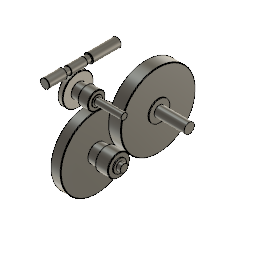
Gearbox Final v12 (Autodesk Fusion 360 design; units mm, degrees)
description: Stage 1
part number: KWG1-R2
description: Layshaft 1
part number: CG1-60R1
description: Stage 2
part number: SSG2-17
description: Layshaft 3
part number: SSG2.5-17
description: Layshaft 2
part number: SSA2-70
description: Stage 3
part number: SS2.5-58
Autodesk Fusion 360 part; units mm, degrees
sketch "Sketch1" plane through (0, 0, 0) normal (0, 1, 0) x (1, 0, 0)
  circle A0 centre (0, 0) radius 9.1
  dimension "d1" = 18.2
  constraint coincident A0.centre origin
  measures "d1" diameter of A0
extrude "Extrude1" add sketch "Sketch1" along normal blind 35 makes body 1
sketch "Sketch2" plane through (0, 35, 0) normal (0, 1, 0) x (-1, 0, 0)
  circle A0 centre (0, 0) radius 9.1
  circle A1 centre (0, 0) radius 6.5
  dimension "d4" = 13
  constraint coincident A0.centre A1.centre
  measures "d4" diameter of A1
extrude "Extrude2" add sketch "Sketch2" along normal blind 10 contours A1 bodies 1
sketch "Sketch3" plane through (0, 45, 0) normal (0, 1, 0) x (-1, 0, 0)
  circle A0 centre (0, 0) radius 6.5
  circle A1 centre (0, 0) radius 8
  dimension "d7" = 16
  constraint coincident A0.centre A1.centre
  measures "d7" diameter of A1
extrude "Extrude3" add sketch "Sketch3" along normal blind 30 contours A0 | A1 bodies 1
sketch "Sketch4" plane through (0, 75, 0) normal (0, 1, 0) x (-1, 0, 0)
  circle A0 centre (0, 0) radius 8
  circle A1 centre (0, 0) radius 6.5
  dimension "d10" = 13
  constraint coincident A0.centre A1.centre
  measures "d10" diameter of A1
extrude "Extrude4" add sketch "Sketch4" along normal blind 10 contours A1 bodies 1
sketch "Sketch5" plane through (0, 85, 0) normal (0, 1, 0) x (-1, 0, 0)
  circle A0 centre (0, 0) radius 6.5
  circle A1 centre (0, 0) radius 9.1
  dimension "d13" = 18.2
  constraint coincident A0.centre A1.centre
  measures "d13" diameter of A1
extrude "Extrude5" add sketch "Sketch5" along normal blind 55 contours A0 | A1 bodies 1
chamfer "Chamfer1" distance 0.5 angle 45 4 edges at (-8.4842, 0, 3.2907) (-8.4842, 35, 3.2907) (8.4842, 85, -3.2907) (8.4842, 140, -3.2907) on bodies 1
sketch "Sketch6" plane through (0, 0, 0) normal (1, 0, 0) x (0, 1, 0)
  circle A0 centre (55, -45) radius 30.06
  circle A1 centre (55, -45) radius 5
  dimension "d17" = 60.12
  dimension "d18" = 10
  constraint concentric A0 A1
  measures "d17" diameter of A0
  measures "d18" diameter of A1
extrude "Extrude6" add sketch "Sketch6" against normal blind 10 separate body makes body 2
sketch "Sketch7" plane through (-10, 0, 0) normal (-1, 0, 0) x (0, -1, 0)
  circle A0 centre (-55, -45) radius 5
  circle A1 centre (-55, -45) radius 30.06
  circle A2 centre (-55, -45) radius 15
  dimension "d21" = 30
  constraint concentric A0 A2
  measures "d21" diameter of A2
extrude "Extrude7" add sketch "Sketch7" along normal blind 10 contours A2 bodies 2
chamfer "Chamfer2" distance 1 angle 45 2 edges at (0, 26.9742, -55.8702) (-10, 26.9742, -34.1298) on bodies 2
chamfer "Chamfer2" distance 0.5 angle 45 3 edges at (0, 50.3384, -43.1919) (-20, 68.9849, -50.4242) (-20, 59.6616, -43.1919) on bodies 2
move_body "Move1" bodies 2 to x (1, 0, 0) y (0, 1, 0) z (0, 0, 1) at (5, 5, 22)
sketch "Sketch8" plane through (5, 0, 0) normal (1, 0, 0) x (0, 1, 0)
  circle A0 centre (60, -23) radius 29.06
  circle A1 centre (60, -23) radius 5.5
  circle A2 centre (60, -23) radius 3
  dimension "d26" = 6
  constraint concentric A0 A2
  measures "d26" diameter of A2
sketch "Sketch11" plane through (0, 0, 0) normal (1, 0, 0) x (0, 1, 0)
  circle A0 centre (0, -50) radius 17
  circle A1 centre (0, -50) radius 6
  dimension "d34" = 34
  dimension "d35" = 12
  constraint concentric A0 A1
  measures "d34" diameter of A0
  measures "d35" diameter of A1
extrude "Extrude10" add sketch "Sketch11" along normal blind 20 separate body makes body 3
sketch "Sketch12" plane through (20, 0, 0) normal (1, 0, 0) x (0, 1, 0)
  circle A0 centre (0, -50) radius 6
  circle A1 centre (0, -50) radius 17
  circle A2 centre (0, -50) radius 14
  dimension "d38" = 28
  constraint concentric A0 A2
  measures "d38" diameter of A2
extrude "Extrude11" add sketch "Sketch12" along normal blind 16 contours A2 bodies 3
chamfer "Chamfer3" distance 0.5 angle 45 3 edges at (36, -13.0526, -55.0626) (36, -5.594, -47.8303) (0, -5.594, -47.8303) on bodies 3
chamfer "Chamfer3" distance 1 angle 45 2 edges at (0, -15.8496, -56.1475) (20, -15.8496, -56.1475) on bodies 3
sketch "Sketch14" plane through (5, 0, 0) normal (1, 0, 0) x (0, 1, 0)
  circle A0 centre (60, -23) radius 29.06
  circle A1 centre (60, -23) radius 5.5
  circle A2 centre (60, -23) radius 5
  dimension "d46" = 10
  constraint concentric A0 A2
  measures "d46" diameter of A2
extrude "Extrude13" add sketch "Sketch14" along normal blind 0 and the other way blind 25 separate body contours A2 makes body 4
sketch "Sketch15" plane through (5, 0, 0) normal (1, 0, 0) x (0, 1, 0)
  circle A0 centre (60, -23) radius 5
  circle A1 centre (60, -23) radius 6
  dimension "d52" = 12
  constraint concentric A0 A1
  measures "d52" diameter of A1
move_body "Move2" bodies 4 to x (1, 0, 0) y (0, 1, 0) z (0, 0, 1) at (43, 0, 0)
sketch "Sketch16" plane through (48, 0, 0) normal (1, 0, 0) x (0, 1, 0)
  circle A0 centre (60, -23) radius 5
  circle A1 centre (60, -23) radius 6
  dimension "d55" = 12
  constraint concentric A0 A1
  measures "d55" diameter of A1
extrude "Extrude15" add sketch "Sketch16" along normal blind 36 contours A0 | A1 bodies 4
move_body "Move3" bodies 4 to x (1, 0, 0) y (0, 1, 0) z (0, 0, 1) at (-43, 0, 0)
move_body "Move4" bodies 3 to x (-1, 0, 0) y (0, 1, 0) z (0, 0, -1) at (41, 60, -73)
sketch "Sketch17" plane through (41, 0, 0) normal (1, 0, 0) x (0, 1, 0)
  circle A0 centre (60, -23) radius 6
  circle A1 centre (60, -23) radius 10
  dimension "d58" = 20
  constraint concentric A0 A1
  measures "d58" diameter of A1
sketch "Sketch18" plane through (0, 0, 0) normal (1, 0, 0) x (0, 1, 0)
  circle A0 centre (0, -150) radius 70
  circle A1 centre (0, -150) radius 9
  dimension "d61" = 140
  dimension "d62" = 18
  constraint concentric A0 A1
  measures "d61" diameter of A0
  measures "d62" diameter of A1
extrude "Extrude17" add sketch "Sketch18" along normal blind 20 separate body makes body 5
move_body "Move5" bodies 5 to x (1, 0, 0) y (0, 1, 0) z (0, 0, 1) at (21, 60, 40)
sketch "Sketch19" plane through (41, 0, 0) normal (1, 0, 0) x (0, 1, 0)
  circle A0 centre (60, -110) radius 9
  circle A1 centre (60, -110) radius 9
  circle A2 centre (60, -110) radius 70
  dimension "d69" = 18
  measures "d69" diameter of A0
extrude "Extrude18" add sketch "Sketch19" along normal blind 0 and the other way blind 30 separate body contours A0 A1 makes body 6
sketch "Sketch20" plane through (0, 0, 0) normal (1, 0, 0) x (0, 1, 0)
  circle A0 centre (0, -300) radius 21.25
  circle A1 centre (0, -300) radius 7.5
  dimension "d74" = 42.5
  dimension "d75" = 15
  constraint concentric A0 A1
  measures "d74" diameter of A0
  measures "d75" diameter of A1
extrude "Extrude19" add sketch "Sketch20" along normal blind 25 separate body makes body 7
sketch "Sketch21" plane through (25, 0, 0) normal (1, 0, 0) x (0, 1, 0)
  circle A0 centre (0, -300) radius 7.5
  circle A1 centre (0, -300) radius 21.25
  circle A2 centre (0, -300) radius 17.5
  dimension "d78" = 35
  constraint concentric A0 A2
  measures "d78" diameter of A2
extrude "Extrude20" add sketch "Sketch21" along normal blind 18 contours A2 bodies 7
chamfer "Chamfer4" distance 0.5 angle 45 3 edges at (0, -6.9925, -297.2879) (43, -16.3157, -306.3283) (43, -6.9925, -297.2879) on bodies 7
chamfer "Chamfer4" distance 1 angle 45 2 edges at (25, -19.812, -307.6843) (0, -19.812, -307.6843) on bodies 7
move_body "Move6" bodies 7 to x (-1, 0, 0) y (0, 1, 0) z (0, 0, -1) at (84, 60, -408.5)
sketch "Sketch22" plane through (0, 0, 0) normal (1, 0, 0) x (0, 1, 0)
  circle A0 centre (0, -325) radius 72.5
  circle A1 centre (0, -325) radius 10
  dimension "d83" = 145
  dimension "d84" = 20
  constraint concentric A0 A1
  measures "d83" diameter of A0
  measures "d84" diameter of A1
extrude "Extrude21" add sketch "Sketch22" along normal blind 25 separate body makes body 8
sketch "Sketch23" plane through (25, 0, 0) normal (1, 0, 0) x (0, 1, 0)
  circle A0 centre (0, -325) radius 10
  circle A1 centre (0, -325) radius 72.5
  circle A2 centre (0, -325) radius 35
  dimension "d87" = 70
  constraint concentric A0 A2
  measures "d87" diameter of A2
extrude "Extrude22" add sketch "Sketch23" along normal blind 12 contours A2 bodies 8
chamfer "Chamfer5" distance 0.5 angle 45 3 edges at (37, -32.6315, -337.6565) (37, -9.3233, -321.3838) (0, -9.3233, -321.3838) on bodies 8
chamfer "Chamfer5" distance 1 angle 45 2 edges at (25, -67.5937, -351.2171) (0, -67.5937, -351.2171) on bodies 8
move_body "Move7" bodies 8 to x (-1, 0, 0) y (0, 1, 0) z (0, 0, -1) at (121, 136.4009, -379.3337)
move_body "Move8" bodies 8 to x (1, 0, 0) y (0, 1, 0) z (0, 0, 1) at (-37, 0, 0)
sketch "Sketch24" plane through (84, 0, 0) normal (1, 0, 0) x (0, 1, 0)
  circle A0 centre (136.4009, -54.3337) radius 10.5
  circle A1 centre (136.4009, -54.3337) radius 71.5
  circle A2 centre (136.4009, -54.3337) radius 10
  dimension "d94" = 20
  constraint concentric A0 A2
  measures "d94" diameter of A2
extrude "Extrude24" add sketch "Sketch24" along normal blind 60 and the other way blind 37 separate body contours A2 makes body 9
move_body "Move9" bodies 6 to x (1, 0, 0) y (0, 1, 0) z (0, 0, 1) at (120, 0, 0)
extrude "Extrude25" cut 1 faces at (131, 62.5872, -107.1538) along direction (1, 0, 0) blind 10 on bodies 6 bodies 6
sketch "Sketch25" plane through (161, 0, 0) normal (1, 0, 0) x (0, 1, 0)
  circle A0 centre (60, -110) radius 9
  circle A1 centre (60, -110) radius 7.5
  dimension "d101" = 15
  constraint concentric A0 A1
  measures "d101" diameter of A1
extrude "Extrude26" add sketch "Sketch25" along normal blind 43 contours A1 bodies 6
sketch "Sketch27" plane through (141, 0, 0) normal (-1, 0, 0) x (0, -1, 0)
  circle A0 centre (-60, -110) radius 9
  circle A1 centre (-60, -110) radius 15
  dimension "d107" = 30
  constraint concentric A0 A1
  measures "d107" diameter of A1
extrude "Extrude28" add sketch "Sketch27" along normal blind 2 contours A0 | A1 bodies 6
move_body "Move10" bodies 7 8 9 to x (1, 0, 0) y (0, 1, 0) z (0, 0, 1) at (0, 0, -1.5)
move_body "Move11" bodies 6 to x (1, 0, 0) y (0, 1, 0) z (0, 0, 1) at (-120, 0, 0)
extrude "Extrude29" add 1 faces at (84, 59.4437, -107.783) along direction (1, 0, 0) blind 10 on bodies 6 bodies 6
sketch "Sketch28" plane through (19, 0, 0) normal (-1, 0, 0) x (0, -1, 0)
  circle A0 centre (-60, -110) radius 15
  circle A1 centre (-60, -110) radius 9
  dimension "d112" = 18
  constraint concentric A0 A1
  measures "d112" diameter of A1
extrude "Extrude30" add sketch "Sketch28" along normal up to surface (39 mm away) contours A1 bodies 6
move_body "Move12" bodies 9 to x (1, 0, 0) y (0, 1, 0) z (0, 0, 1) at (95, 0, 0)
sketch "Sketch29" plane through (142, 0, 0) normal (-1, 0, 0) x (0, -1, 0)
  circle A0 centre (-136.4009, -55.8337) radius 10
  circle A1 centre (-136.4009, -55.8337) radius 15
  dimension "d115" = 30
  constraint concentric A0 A1
  measures "d115" diameter of A1
extrude "Extrude31" add sketch "Sketch29" along normal blind 2 contours A0 | A1 bodies 9
move_body "Move13" bodies 9 to x (1, 0, 0) y (0, 1, 0) z (0, 0, 1) at (-95, 0, 0)
move_body "Move14" bodies 4 to x (1, 0, 0) y (0, 1, 0) z (0, 0, 1) at (130, 0, 0)
sketch "Sketch30" plane through (171, 0, 0) normal (1, 0, 0) x (0, 1, 0)
  circle A0 centre (60, -23) radius 6
  circle A1 centre (60, -23) radius 10
  dimension "d119" = 20
  constraint concentric A0 A1
  measures "d119" diameter of A1
extrude "Extrude32" add sketch "Sketch30" along normal blind 1 contours A0 | A1 bodies 4
move_body "Move15" bodies 4 to x (1, 0, 0) y (0, 1, 0) z (0, 0, 1) at (-130, 0, 0)
sketch "Sketch32" plane through (42, 0, 0) normal (1, 0, 0) x (0, 1, 0)
  circle A0 centre (60, -23) radius 10
  circle A1 centre (60, -23) radius 6
  dimension "d123" = 12
  constraint concentric A0 A1
  measures "d123" diameter of A1
extrude "Extrude33" add sketch "Sketch32" along normal up to surface (52 mm away) contours A1 bodies 4
sketch "Sketch33" plane through (84, 0, 0) normal (1, 0, 0) x (0, 1, 0)
  circle A0 centre (136.4009, -55.8337) radius 10.5
  circle A1 centre (136.4009, -55.8337) radius 71.5
  circle A2 centre (136.4009, -55.8337) radius 20
  circle A3 centre (136.4009, -55.8337) radius 10
  dimension "d126" = 40
  dimension "d127" = 20
  constraint concentric A0 A2
  constraint concentric A2 A3
  measures "d126" diameter of A2
  measures "d127" diameter of A3
extrude "Extrude34" add sketch "Sketch33" along normal blind 2 separate body contours A0 | A2 makes body 10
sketch "Sketch34" plane through (84, 0, 0) normal (1, 0, 0) x (0, 1, 0)
  circle A0 centre (60, -110) radius 8
  circle A1 centre (60, -110) radius 20.25
  circle A2 centre (60, -110) radius 12.5
  circle A3 centre (60, -110) radius 7.5
  dimension "d130" = 25
  dimension "d131" = 15
  constraint concentric A0 A2
  constraint concentric A2 A3
  measures "d130" diameter of A2
  measures "d131" diameter of A3
extrude "Extrude35" add sketch "Sketch34" along normal blind 2 separate body contours A0 | A2 makes body 11
sketch "Sketch35" plane through (-15, 0, 0) normal (-1, 0, 0) x (0, -1, 0)
  circle A0 centre (-60, -23) radius 14.5
  circle A1 centre (-60, -23) radius 5.5
  circle A2 centre (-60, -23) radius 10
  circle A3 centre (-60, -23) radius 5
  dimension "d134" = 20
  dimension "d135" = 10
  constraint concentric A0 A2
  constraint concentric A2 A3
  measures "d134" diameter of A2
  measures "d135" diameter of A3
extrude "Extrude36" add sketch "Sketch35" along normal blind 1 separate body contours A1 | A2 makes body 12
move_body "Move16" bodies 1 to x (1, 0, 0) y (0, 1, 0) z (0, 0, 1) at (0, 0, 15)
copy_body "Body->Comp1" bodies 1 removing the originals makes body 13 in component "Worm "
copy_body "Body->Comp2" bodies 12 removing the originals makes body 14 in component "Fixing "
copy_body "Body->Comp3" bodies 2 removing the originals makes body 15 in component "Wheel"
copy_body "Body->Comp4" bodies 3 removing the originals makes body 16 in component "Spur 17 M2"
copy_body "Body->Comp5" bodies 4 removing the originals makes body 17 in component "Layshaft 1"
copy_body "Body->Comp6" bodies 10 removing the originals makes body 18 in component "Fixing 3"
copy_body "Body->Comp7" bodies 9 removing the originals makes body 19 in component "Layshaft 3"
copy_body "Body->Comp8" bodies 7 removing the originals makes body 20 in component "Spur 17 M2.5"
copy_body "Body->Comp9" bodies 11 removing the originals makes body 21 in component "Fixing 2"
copy_body "Body->Comp10" bodies 5 removing the originals makes body 22 in component "Spur 70 M2"
copy_body "Body->Comp11" bodies 8 removing the originals makes body 23 in component "Spur 58 M2.5"
copy_body "Body->Comp12" bodies 6 removing the originals makes body 24 in component "Layshaft 2"
chamfer "Chamfer1'" distance 1 angle 45 2 edges at (41, -5.2629, -135.3131) (21, -5.2629, -135.3131) on bodies 22 in component "Spur 70 M2"
component "Worm " placed x (1, 0, 0) y (0, 1, 0) z (0, 0, 1) at (0, 0, 0)
component "Fixing " placed x (1, 0, 0) y (0, 1, 0) z (0, 0, 1) at (0, 0, 0)
component "Wheel" placed x (1, 0, 0) y (0, 1, 0) z (0, 0, 1) at (0, 0, 0)
component "Spur 17 M2" placed x (1, 0, 0) y (0, 1, 0) z (0, 0, 1) at (0, 0, 0)
component "Layshaft 1" placed x (1, 0, 0) y (0, 1, 0) z (0, 0, 1) at (0, 0, 0)
component "Fixing 3" placed x (1, 0, 0) y (0, 1, 0) z (0, 0, 1) at (0, 0, 0)
component "Layshaft 3" placed x (1, 0, 0) y (0, 1, 0) z (0, 0, 1) at (0, 0, 0)
component "Spur 17 M2.5" placed x (1, 0, 0) y (0, 1, 0) z (0, 0, 1) at (0, 0, 0)
component "Fixing 2" placed x (1, 0, 0) y (0, 1, 0) z (0, 0, 1) at (0, 0, 0)
component "Spur 70 M2" placed x (1, 0, 0) y (0, 1, 0) z (0, 0, 1) at (0, 0, 0)
component "Spur 58 M2.5" placed x (1, 0, 0) y (0, 1, 0) z (0, 0, 1) at (0, 0, 0)
component "Layshaft 2" placed x (1, 0, 0) y (0, 1, 0) z (0, 0, 1) at (0, 0, 0)
named bodies: "Worm", "Wheel", "Spur 17 M2", "Layshaft 1", "Spur 70 M2", "Layshaft 2", "Spur 17 M2.5", "Spur 58 M2.5", "Layshaft 3", "Fixing 3", "Fixing 2", "Fixing 1"
